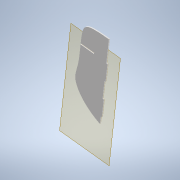
# Autodesk Inventor part: поперечная_поддержка
Saved by Autodesk Inventor 2020 (Build 240168000, 168)
## iProperties
Created: 2022-03-08
Part Number: поперечная_поддержка
Material: Типовые
Document SubType Name: Modeling
Designer: Администратор
Density: 1 g/cm^3
Appearance: По умолчанию
Author: Администратор
Autodesk Inventor part; units mm, degrees
ref_plane "YZ Plane" through (0, 0, 0) normal (1, 0, 0) x (0, 1, 0)
ref_plane "XZ Plane" through (0, 0, 0) normal (0, 1, 0) x (-1, 0, 0)
ref_plane "XY Plane" through (0, 0, 0) normal (0, 0, 1) x (1, 0, 0)
ref_plane "РабПлоскость1" through (-13.5579, -94.7398, 0) normal (0, 0, 1) x (0.9934395, -0.1143588, 0)
sketch "Эскиз1" plane through (-13.5579, -94.7398, 0) normal (0, 0, 1) x (0.9934395, -0.1143588, 0)
  line L0 (25.9016, 248.6307) -> (-44.0832, 248.6307) construction
  line L1 (-44.0832, 248.6307) -> (-55.2417, 234.7693) construction
  line L2 (-55.2417, 234.7693) -> (-68.4885, 234.7693) construction
  line L3 (-68.4885, 234.7693) -> (-68.4885, 175.7756) construction
  line L4 (-68.4885, 175.7756) -> (-68.4885, 136.8397) construction
  line L5 (-68.4885, 136.8397) -> (-68.4885, 100.2635) construction
  line L6 (-68.4885, 100.2635) -> (-79.6973, 58.9679) construction
  line L7 (-79.6973, 58.9679) -> (-72.618, 32.4207) construction
  line L8 (-72.618, 32.4207) -> (-26.2068, -16.2312) construction
  line L9 (-26.2068, -16.2312) -> (25.9016, -35.7278) construction
  spline S0 degree 4 poles (25.9016, 248.6307) (-44.0832, 248.6307) (-55.2417, 234.7693) (-68.4885, 234.7693) (-68.4885, 175.7756) (-68.4885, 136.8397) (-68.4885, 100.2635) (-79.6973, 58.9679) (-72.618, 32.4207) (-26.2068, -16.2312) (25.9016, -35.7278) knots 1 1 1 1 1 2 3 4 5 6 7 8 8 8 8 8
  line L10 (25.9016, 248.6307) -> (25.9016, -35.7278)
  line L11 (29.9016, 248.6307) -> (25.9016, 248.6307) projected
  line L12 (25.9016, 248.6307) -> (325.9016, 248.6307) construction
  line L13 (25.9016, 248.6307) -> (-360.9302, 248.6307)
  line L14 (29.9016, -35.7278) -> (25.9016, -35.7278) projected
  line L15 (25.9016, -35.7278) -> (-58.0724, -35.7278)
  point P0 (2.6346, 95.6688)
  constraints: 8 end point, 4 horizontal, 4 vertical, 1 point on line, 3 other
extrude "Выдавливание1" add sketch "Эскиз1" along normal mid plane 4
sketch "Эскиз2" plane through (10.9482, -108.3491, 1.5) normal (0.9934395, -0.1143588, 0) x (0, 0, -1)
  line L0 (3, 0) -> (0, 0) projected
  line L1 (0, 0) -> (0, 59.7017)
  line L2 (-0.5, -25.0103) -> (-0.5, 259.3482) projected
  line L3 (3.5, 259.3482) -> (3.5, -25.0103) projected
  line L4 (3, 59.7017) -> (3, 119.4034)
  line L5 (0, 119.4034) -> (0, 179.1051)
  line L6 (0, 179.1051) -> (3, 179.1051)
  line L7 (3, 179.1051) -> (3, 238.8068)
  line L8 (0, 238.8068) -> (0, 298.5085)
  line L9 (0, 298.5085) -> (3, 298.5085) projected
  line L10 (0, 59.7017) -> (3, 59.7017)
  line L11 (3, 119.4034) -> (0, 119.4034)
  line L12 (3, 238.8068) -> (0, 238.8068)
  line L13 (0, 59.7017) -> (0, 119.4034)
  line L14 (0, 179.1051) -> (0, 238.8068)
  line L15 (3, 238.8068) -> (3, 298.5085)
  line L16 (0, 298.5085) -> (3, 298.5085)
  line L17 (0, 0) -> (3, 0)
  line L18 (3, 59.7017) -> (3, 0)
  line L19 (3, 59.7017) -> (0, 59.7017)
  line L20 (0, 119.4034) -> (3, 119.4034)
  line L21 (0, 59.7017) -> (0, 119.4034)
  line L22 (3, 179.1051) -> (0, 179.1051)
  line L23 (0, 238.8068) -> (3, 238.8068)
  line L24 (3, 238.8068) -> (3, 298.5085)
  line L25 (0, 298.5085) -> (3, 298.5085)
  line L26 (0, 238.8068) -> (0, 298.5085)
  line L27 (3, 179.1051) -> (3.5, 179.1051)
  line L28 (3, 119.4034) -> (3.5, 119.4034)
  line L29 (3.5, 179.1051) -> (3.5, 119.4034)
  line L30 (0, 179.1051) -> (-0.5, 179.1051)
  line L31 (-0.5, 179.1051) -> (-0.5, 119.4034)
  line L32 (0, 119.4034) -> (-0.5, 119.4034)
  line L33 (3, 59.7017) -> (3.5, 59.7017)
  line L34 (3.5, 59.7017) -> (3.5, 0)
  line L35 (3, 0) -> (3.5, 0)
  line L36 (0, 0) -> (-0.5, 0)
  line L37 (-0.5, 0) -> (-0.5, 59.7017)
  line L38 (-0.5, 59.7017) -> (0, 59.7017)
  point P0 (1.5, 106.3863)
  point P1 (-0.5, 259.3482)
  point P2 (3.5, -25.0103)
  point P3 (3, 59.7017)
  constraints: 68 end point, 9 point on line, 7 perpendicular, 7 vertical, 6 horizontal, 4 parallel, 3 collinear, 18 other
extrude "Выдавливание2" add sketch "Эскиз2" along normal blind 4 contours L0 L1 L10 L18 | L18 L33 L3 L35 | L36 L2 L38 L1 | L11 L5 L6 L27 L3 L28 | L32 L2 L30 L5
sketch "Эскиз3" plane through (-13.5579, -94.7398, 0) normal (0, 0, 1) x (0.9934395, -0.1143588, 0)
  point P0 (2.6346, 95.6688)
sketch "Эскиз4" plane through (-13.5579, -94.7398, 0) normal (0, 0, 1) x (0.9934395, -0.1143588, 0)
  line L0 (-21.9452, -13.2655) -> (34.011, -13.2655) projected
  line L1 (-21.9452, -13.2655) -> (34.011, -13.2655) projected
  line L2 (34.011, -13.2655) -> (34.011, -16.2655) projected
  line L3 (-21.9452, -13.2655) -> (34.011, -13.2655) projected
  line L4 (-21.9452, -16.2655) -> (-21.9452, -13.2655) projected
  line L5 (34.011, -16.2655) -> (-21.9452, -16.2655) projected
  line L6 (-21.9452, -16.2655) -> (-21.9452, -13.2655)
  line L7 (-69.5874, -16.2655) -> (-21.9452, -16.2655)
  line L8 (-21.9452, -13.2655) -> (-69.5874, -13.2655)
  line L9 (-69.5874, -13.2655) -> (-69.5874, -16.2655)
  line L10 (-21.9452, -13.2655) -> (-21.9452, -12.7655)
  line L11 (-21.9452, -12.7655) -> (-69.5874, -12.7655)
  line L12 (-69.5874, -12.7655) -> (-69.5874, -13.2655)
  line L13 (-69.5874, -16.2655) -> (-69.5874, -16.7655)
  line L14 (-69.5874, -16.7655) -> (-21.9452, -16.7655)
  line L15 (-21.9452, -16.7655) -> (-21.9452, -16.2655)
  point P0 (2.6346, 95.6688)
  point P1 (-66.0194, -13.2655)
  dimension "d16" = 0.5
  dimension "d17" = 0.5
  constraints: 20 end point, 4 perpendicular, 3 point on line, 2 collinear, 1 coincident, 1 horizontal, 1 parallel, 1 vertical
  measures "d16" distance of L0.start L10.end
  measures "d17" distance of L7.start L13.end
extrude "Выдавливание3" cut sketch "Эскиз4" against normal through all both and the other way through all contours L4 L7 L9 L8 | L8 L12 L11 L10 | L15 L14 L13 L7
sketch "Эскиз5" plane through (-13.5579, -94.7398, 0) normal (0, 0, 1) x (0.9934395, -0.1143588, 0)
  line L0 (25.9016, 173.347) -> (25.9016, 169.347) projected
  line L1 (-19.0984, 173.347) -> (25.9016, 173.347) projected
  line L2 (-19.0984, 173.347) -> (-19.0984, 169.347) projected
  line L3 (25.9016, 169.347) -> (-19.0984, 169.347) projected
  line L4 (-19.0984, 173.347) -> (-19.0984, 169.347)
  line L5 (-78.4724, 173.347) -> (-19.0984, 173.347)
  line L6 (-78.4724, 173.347) -> (-78.4724, 169.347)
  line L7 (-78.4724, 169.347) -> (-19.0984, 169.347)
  line L8 (-19.0984, 173.347) -> (-19.0984, 169.347)
  line L9 (-78.4724, 173.347) -> (-78.4724, 173.847)
  line L10 (-78.4724, 173.847) -> (-19.0984, 173.847)
  line L11 (-19.0984, 173.847) -> (-19.0984, 173.347)
  line L12 (-19.0984, 169.347) -> (-19.0984, 168.847)
  line L13 (-19.0984, 168.847) -> (-78.4724, 168.847)
  line L14 (-78.4724, 168.847) -> (-78.4724, 169.347)
  point P0 (2.6346, 95.6688)
  dimension "d14" = 0.5
  dimension "d15" = 0.5
  constraints: 22 end point, 4 perpendicular, 4 vertical, 2 collinear, 1 parallel
  measures "d14" distance of L5.start L9.end
  measures "d15" distance of L2.end L12.end
extrude "Выдавливание4" cut sketch "Эскиз5" along normal through all both and the other way through all contours L2 L7 L6 L5 | L5 L9 L10 L11 | L12 L13 L14 L7
sketch "Эскиз6" plane through (-13.5579, -94.7398, -2) normal (0, 0, -1) x (-0.9934395, 0.1143588, 0)
  line L0 (16.8024, -31.0891) -> (36.8024, -31.0891)
  line L1 (36.8024, -31.0891) -> (36.8024, -46.0891)
  line L2 (36.8024, -46.0891) -> (16.8024, -46.0891)
  line L3 (16.8024, -46.0891) -> (16.8024, -31.0891)
  point P0 (-2.6346, 95.6688)
  dimension "d10" = 20
  dimension "d11" = 15
  constraints: 8 end point, 3 perpendicular, 1 horizontal
  measures "d10" distance of L0.start L0.end
  measures "d11" distance of L0.end L1.end
extrude "Выдавливание5" cut sketch "Эскиз6" against normal through all
